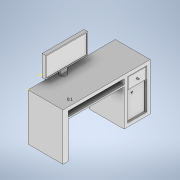
# Autodesk Inventor part: desk
Saved by Autodesk Inventor 2022 (Build 260153000, 153)
## iProperties
Created: 2023-05-02
Part Number: desk
Material: Generic
Document SubType Name: Modeling
Designer: mihir
Density: 1 g/cm^3
Appearance: Default
Author: mihir
Autodesk Inventor part; units mm, degrees
ref_plane "YZ Plane" through (0, 0, 0) normal (1, 0, 0) x (0, 1, 0)
ref_plane "XZ Plane" through (0, 0, 0) normal (0, 1, 0) x (-1, 0, 0)
ref_plane "XY Plane" through (0, 0, 0) normal (0, 0, 1) x (1, 0, 0)
sketch "Sketch1" plane through (0, 0, 0) normal (0, 0, 1) x (1, 0, 0)
  line L0 (0, 0) -> (25, 0)
  line L1 (25, 0) -> (25, 10)
  line L2 (25, 10) -> (0, 10)
  line L3 (0, 10) -> (0, 0)
  dimension "d0" = 25
  dimension "d1" = 10
  constraints: 8 end point, 2 parallel, 1 horizontal, 1 perpendicular
  measures "d0" distance of L2.end L1.end
  measures "d1" distance of L1.end L0.end
extrude "Extrusion1" add sketch "Sketch1" along normal blind 1
sketch "Sketch2" plane through (0, 0, 1) normal (0, 0, 1) x (1, 0, 0)
  line L0 (25, 10) -> (0, 10) projected
  line L1 (0, 10) -> (1.5, 10)
  line L2 (1.5, 10) -> (1.5, 0)
  line L3 (1.5, 0) -> (0, 0)
  line L4 (0, 0) -> (0, 10)
  line L5 (25, 0) -> (25, 10) projected
  line L6 (25, 10) -> (17.5, 10)
  line L7 (17.5, 10) -> (17.5, 0)
  line L8 (17.5, 0) -> (25, 0)
  line L9 (25, 0) -> (25, 10)
  line L10 (0, 0) -> (25, 0) projected
  line L11 (0, 0) -> (25, 0)
  line L12 (25, 0) -> (25, 1)
  line L13 (25, 1) -> (0, 1)
  line L14 (0, 1) -> (0, 0)
  point P0 (1.5, 1)
  point P1 (17.5, 1)
  dimension "d4" = 1.5
  dimension "d5" = 10
  dimension "d6" = 7.5
  dimension "d7" = 10
  dimension "d8" = 25
  dimension "d9" = 1
  constraints: 24 end point, 6 parallel, 3 horizontal, 3 perpendicular
  measures "d4" distance of L2.end L3.end
  measures "d5" distance of L1.end L2.end
  measures "d6" distance of L8.end L7.end
  measures "d7" distance of L7.end L6.end
  measures "d8" distance of L13.end L12.end
  measures "d9" distance of L12.end L11.end
extrude "Extrusion2" add sketch "Sketch2" along normal blind 2 contours L5 L8 L7 L13 | L7 L10 L2 L13 | L2 L3 L4 L13
extrude "Extrusion3" add sketch "Sketch2" along normal blind 12.5 contours L5 L13 L7 L0 | L5 L8 L7 L13 | L2 L13 L4 L0 | L2 L3 L4 L13
sketch "Sketch3" plane through (1.5, 1, 1) normal (0, 1, 0) x (1, 0, 0)
  line L0 (7, 0) -> (9, 0)
  line L1 (9, 0) -> (9, -0.5)
  line L2 (9, -0.5) -> (7, -0.5)
  line L3 (7, -0.5) -> (7, 0)
  line L4 (16, 0) -> (0, 0) projected
  line L5 (0, 0) -> (0, -12.5) projected
  point P0 (-1.5, 1)
  dimension "d16" = 2
  dimension "d17" = 0.5
  dimension "d18" = 0
  dimension "d19" = 7
  constraints: 8 end point, 2 parallel, 1 horizontal, 1 perpendicular
  measures "d16" distance of L1.end L2.end
  measures "d17" distance of L0.end L1.end
  measures "d18" distance between parallel lines of L4 L0
  measures "d19" distance between parallel lines of L5 L3
extrude "Extrusion5" cut sketch "Sketch3" against normal through all
fillet "Fillet1" radius 0.1 2 edges at (10.5, 0.5, 1.5) (8.5, 0.5, 1.5)
shell "Shell1" thickness 1 removed faces 1 at (22.5, 10, 4.8333)
sketch "Sketch4" plane through (18.5, 1, 12.5) normal (0, 1, 0) x (1, 0, 0)
  line L0 (0.25, 8) -> (5.25, 8)
  line L1 (5.25, 8) -> (5.25, 0)
  line L2 (5.25, 0) -> (0.25, 0)
  line L3 (0.25, 0) -> (0.25, 8)
  line L4 (0, 0) -> (0, 11.5) projected
  line L5 (5.5, 0) -> (0, 0) projected
  point P0 (-18.5, 12.5)
  dimension "d24" = 5
  dimension "d25" = 0.25
  dimension "d26" = 0
  dimension "d27" = 8
  constraints: 8 end point, 2 parallel, 1 horizontal, 1 perpendicular
  measures "d24" distance of L0.start L0.end
  measures "d25" distance between parallel lines of L4 L3
  measures "d26" distance between parallel lines of L5 L2
  measures "d27" distance between parallel lines of L2 L0
extrude "Extrusion6" add sketch "Sketch4" along normal blind 8.5
sketch "Sketch5" plane through (18.5, 9.5, 12.5) normal (0, 1, 0) x (1, 0, 0)
  circle A0 centre (1.75, 6.5) radius 0.25
  line L0 (5.25, 8) -> (0.25, 8) projected
  line L1 (0.25, 8) -> (0.25, 0) projected
  point P0 (-18.5, 12.5)
  dimension "d30" = 0.5
  dimension "d31" = 1.5
  dimension "d32" = 1.5
  constraints: 1 centre point
  measures "d30" diameter of A0
  measures "d31" distance from line of L0 A0.centre
  measures "d32" distance from line of L1 A0.centre
extrude "Extrusion7" add sketch "Sketch5" along normal blind 0.1
fillet "Fillet2" radius 0.05 1 edges at (20, 9.6, 6)
sketch "Sketch6" plane through (18.5, 1, 1) normal (0, 1, 0) x (1, 0, 0)
  line L0 (0.05, -0.05) -> (5.45, -0.05)
  line L1 (5.45, -0.05) -> (5.45, -3.45)
  line L2 (5.45, -3.45) -> (0.05, -3.45)
  line L3 (0.05, -3.45) -> (0.05, -0.05)
  line L4 (0, -11.5) -> (0, 0) projected
  line L5 (0, 0) -> (5.5, 0) projected
  point P0 (-18.5, 1)
  dimension "d36" = 5.4
  dimension "d37" = 0.05
  dimension "d38" = 0.05
  dimension "d39" = 3.4
  constraints: 8 end point, 2 parallel, 1 horizontal, 1 perpendicular
  measures "d36" distance of L0.start L0.end
  measures "d37" distance between parallel lines of L4 L3
  measures "d38" distance between parallel lines of L5 L0
  measures "d39" distance between parallel lines of L0 L2
extrude "Extrusion8" add sketch "Sketch6" along normal blind 9
fillet "Fillet3" radius 0.15 4 edges at (18.55, 10, 2.75) (21.25, 10, 1.05) (21.25, 10, 4.45) (23.95, 10, 2.75)
sketch "Sketch7" plane through (18.5, 10, 1) normal (0, 1, 0) x (1, 0, 0)
  circle A0 centre (2.75, -1.75) radius 0.15
  line L0 (0.2, -0.2) -> (5.3, -0.2) projected
  line L1 (0.2, -3.3) -> (0.2, -0.2) projected
  point P0 (-18.5, 1)
  dimension "d43" = 0.3
  dimension "d44" = 1.55
  dimension "d45" = 2.55
  constraints: 1 centre point
  measures "d43" diameter of A0
  measures "d44" distance from line of L0 A0.centre
  measures "d45" distance from line of L1 A0.centre
ref_plane "Work Plane1" through (18.5, 10.5, 1) normal (0, 1, 0) x (1, 0, 0)
sketch "Sketch8" plane through (18.5, 10.5, 1) normal (0, 1, 0) x (1, 0, 0)
  circle A0 centre (2.75, -1.75) radius 0.25
  point P0 (-18.5, 1)
  dimension "d47" = 0.5
  constraints: 1 centre point, 1 coincident
  measures "d47" diameter of A0
loft "Loft1" add profiles "Sketch7", "Sketch8"
fillet "Fillet4" radius 0.075 1 edges at (21, 10.5, 2.75)
fillet "Fillet5" radius 0.075 1 edges at (21.1, 10, 2.75)
sketch "Sketch9" plane through (0, 0, 0) normal (0, -1, 0) x (1, 0, 0)
  point P0 (0, 0)
ref_plane "Work Plane2" through (0, 1, 0) normal (0, -1, 0) x (1, 0, 0)
sketch "Sketch10" plane through (0, 1, 0) normal (0, -1, 0) x (1, 0, 0)
  line L0 (3, -8) -> (15, -8)
  line L1 (15, -8) -> (15, -2)
  line L2 (15, -2) -> (3, -2)
  line L3 (3, -2) -> (3, -8)
  line L4 (25, 0) -> (0, 0) projected
  line L5 (0, 0) -> (0, 13.5) projected
  line L6 (14.75, -7.75) -> (3.25, -7.75)
  line L7 (3.25, -7.75) -> (3.25, -2.25)
  line L8 (3.25, -2.25) -> (14.75, -2.25)
  line L9 (14.75, -2.25) -> (14.75, -7.75)
  dimension "d55" = 12
  dimension "d56" = 6
  dimension "d57" = 2
  dimension "d58" = 3
  dimension "d59" = 0.25
  constraints: 16 end point, 4 parallel, 2 perpendicular, 1 horizontal, 3 other
  measures "d55" distance of L2.end L1.end
  measures "d56" distance of L1.end L0.end
  measures "d57" distance between parallel lines of L2 L4
  measures "d58" distance between parallel lines of L5 L3
  measures "d59" distance between parallel lines of L0 L6
extrude "Extrusion9" add sketch "Sketch10" against normal blind 1
extrude "Extrusion10" add sketch "Sketch10" against normal blind 0.9 contours L6 L7 L8 L9
sketch "Sketch11" plane through (0, 0, 0) normal (0, 0, -1) x (-1, 0, 0)
  line L0 (-15, 1) -> (-3, 1) projected
  circle A0 centre (-9, 1) radius 1
  line L1 (-10.5, 0) -> (-8.5, 0) projected
  point P0 (0, 0)
  constraints: 1 centre point, 1 midpoint, 1 tangent
extrude "Extrusion11" add sketch "Sketch11" along normal blind 3.5
sketch "Sketch12" plane through (0, 0, 0) normal (-1, 0, 0) x (0, 0, 1)
  line L0 (-2, 1) -> (-2, 2) projected
  line L1 (-2, 2) -> (-0.25, 2)
  line L2 (-0.25, 2) -> (-0.25, 1.25)
  line L3 (-0.25, 1.25) -> (-2, 1.25)
  line L4 (-2, 1.25) -> (-2, 2)
  line L5 (0, 0) -> (-3.5, 0) projected
  line L6 (-2, 0) -> (-0.25, 0)
  line L7 (-0.25, 0) -> (-0.25, 0.75)
  line L8 (-0.25, 0.75) -> (-2, 0.75)
  line L9 (-2, 0.75) -> (-2, 0)
  dimension "d66" = 1.75
  dimension "d67" = 0.75
  dimension "d68" = 1.75
  dimension "d69" = 0.75
  constraints: 16 end point, 4 parallel, 2 horizontal, 2 perpendicular, 1 point on line
  measures "d66" distance of L2.end L3.end
  measures "d67" distance of L1.end L2.end
  measures "d68" distance of L8.end L7.end
  measures "d69" distance of L7.end L6.end
extrude "Extrusion12" cut sketch "Sketch12" against normal through all
sketch "Sketch13" plane through (0, 0, -3.5) normal (0, 0, -1) x (-1, 0, 0)
  arc A0 (-8.5641, 1.9) -> (-9.4359, 1.9) centre (-9, 1) ccw projected
  line L0 (-8.5641, 1.9) -> (-9.4359, 1.9) projected
  point P0 (0, 0)
extrude "Extrusion13" cut sketch "Sketch13" against normal up to surface (1.25 mm away)
sketch "Sketch14" plane through (1.5, 0, 3) normal (0, -1, 0) x (1, 0, 0)
  line L0 (22.5, 9.5) -> (17, 9.5) projected
  line L1 (21, 9) -> (18.5, 9)
  line L2 (18.5, 9) -> (18.5, 9.5)
  line L3 (18.5, 9.5) -> (21, 9.5)
  line L4 (21, 9.5) -> (21, 9)
  line L5 (23.5, -3) -> (23.5, 10.5) projected
  point P0 (-1.5, -3)
  dimension "d74" = 2.5
  dimension "d75" = 2.5
  dimension "d76" = 0.5
  constraints: 8 end point, 2 parallel, 1 horizontal, 1 perpendicular, 1 point on line
  measures "d74" distance of L1.start L1.end
  measures "d75" distance between parallel lines of L5 L4
  measures "d76" distance between parallel lines of L0 L1
extrude "Extrusion14" cut sketch "Sketch14" against normal blind 1
sketch "Sketch15" plane through (1.5, 1, 3) normal (0, 1, 0) x (1, 0, 0)
  line L0 (0, 0) -> (0, -10.5) projected
  line L1 (0, 0) -> (16, 0)
  line L2 (16, 0) -> (16, 0.5)
  line L3 (16, 0.5) -> (0, 0.5)
  line L4 (0, 0.5) -> (0, 0)
  point P0 (-1.5, 3)
  dimension "d79" = 16
  dimension "d80" = 0.5
  constraints: 8 end point, 2 parallel, 1 horizontal, 1 perpendicular
  measures "d79" distance of L3.end L2.end
  measures "d80" distance of L2.end L1.end
extrude "Extrusion15" add sketch "Sketch15" along normal up to surface (9 mm away)
sketch "Sketch16" plane through (1.5, 0, 3) normal (0, -1, 0) x (1, 0, 0)
  line L0 (22.5, 9.5) -> (17, 9.5) projected
  line L1 (19.1767, 9.5) -> (15.2446, 9.1939) construction
  line L2 (15.2446, 9.1939) -> (13.3006, 8.1336) construction
  line L3 (13.3006, 8.1336) -> (11.1737, 6.9735) construction
  line L4 (11.1737, 6.9735) -> (8.8892, 4.7275) construction
  line L5 (8.8892, 4.7275) -> (7.4687, 2.4784) construction
  line L6 (7.4687, 2.4784) -> (5.348, -0.8793) construction
  line L7 (6.5, -5) -> (1.5, -5) projected
  line L8 (5.348, -0.8793) -> (3.4924, -5) construction
  spline S0 degree 4 poles (19.1767, 9.5) (15.2446, 9.1939) (13.3006, 8.1336) (11.1737, 6.9735) (8.8892, 4.7275) (7.4687, 2.4784) (5.348, -0.8793) (3.4924, -5) knots 1 1 1 1 1 2 3 4 5 5 5 5 5
  line L9 (19.1844, 9.4003) -> (19.1767, 9.5)
  spline S1 degree 5 poles (19.1844, 9.4003) (18.2428, 9.328) (17.3025, 9.2266) (16.3687, 9.0993) (15.0308, 8.827) (13.7913, 8.2774) (13.4334, 8.0817) (12.7939, 7.7115) (12.1658, 7.3222) (11.8888, 7.1396) (11.3549, 6.768) (10.8463, 6.3625) (10.6036, 6.1558) (10.1253, 5.7184) (9.6767, 5.2505) (9.4567, 5.0051) (8.992, 4.4539) (8.5604, 3.8762) (8.3337, 3.557) (7.779, 2.7463) (7.2448, 1.922) (6.9288, 1.4228) (5.992, -0.1276) (5.1424, -1.7284) (4.6038, -2.8239) (4.0844, -3.9282) (3.5836, -5.0411) knots 0 0 0 0 0 0 0.20833 0.20833 0.20833 0.298158 0.298158 0.298158 0.37131 0.37131 0.37131 0.441556 0.441556 0.441556 0.5142 0.5142 0.5142 0.600534 0.600534 0.600534 0.730841 0.730841 0.730841 1 1 1 1 1 1
  point P0 (-1.5, -3)
  dimension "d83" = 0.1
  constraints: 2 end point, 2 point on line, 1 perpendicular, 6 other
body "Solid1"
